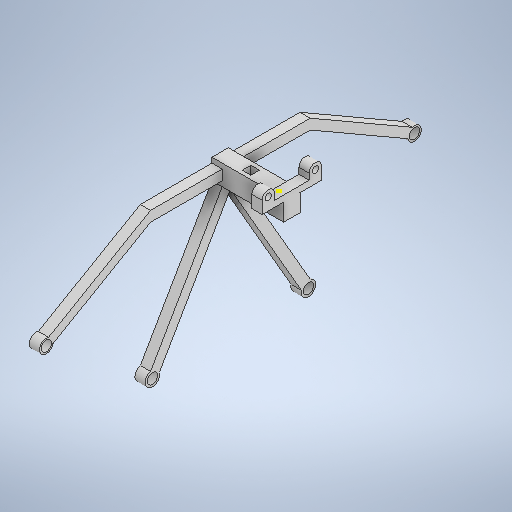
# Autodesk Inventor part: Pelvis proto1
Saved by Autodesk Inventor 2025.1 (Build 291241020, 241B)
## iProperties
Created: 2024-10-22
Part Number: Pelvis proto1
Material: Generic
Document SubType Name: Modeling
Designer: morte
Density: 1 g/cm^3
Appearance: Default
Author: morte
Autodesk Inventor part; units mm, degrees
ref_plane "YZ Plane" through (0, 0, 0) normal (1, 0, 0) x (0, 1, 0)
sketch "Sketch1" plane through (0, 0, 0) normal (1, 0, 0) x (0, 1, 0)
  line L0 (0, 0) -> (0, 8.5)
  line L1 (0, 14.5) -> (6, 14.5)
  line L2 (0, 0) -> (0, -8.5)
  line L3 (0, -14.5) -> (6, -14.5)
  line L4 (6, -14.5) -> (6, -8.5)
  line L5 (6, -8.5) -> (0, -8.5)
  line L6 (6, 14.5) -> (6, 8.5)
  line L7 (6, 8.5) -> (0, 8.5)
  line L8 (0, 14.5) -> (-3, 14.5)
  line L9 (-3, 14.5) -> (-3, -14.5)
  line L10 (-3, -14.5) -> (0, -14.5)
  line L11 (0, -8.5) -> (-3, -8.5)
  line L12 (0, 8.5) -> (-3, 8.5)
  line L13 (-3, 0) -> (-3, -5)
  dimension "d0" = 14.5
  dimension "d1" = 6
  dimension "d2" = 14.5
  dimension "d3" = 6
  dimension "d4" = 90
  dimension "d5" = 29
  dimension "d6" = 6
  dimension "d7" = 6
  dimension "d8" = 3
  dimension "d9" = 5
  constraints: 28 end point, 7 perpendicular, 4 point on line, 3 vertical, 1 collinear, 1 horizontal, 1 midpoint
  measures "d0" distance of L0.start L1.start
  measures "d1" distance of L1.start L1.end
  measures "d2" distance of L0.start L3.start
  measures "d3" distance of L3.start L3.end
  measures "d4" angle of L3 L2
  measures "d5" distance of L3.start L1.start
  measures "d6" distance of L3.end L4.end
  measures "d7" distance of L1.end L6.end
  measures "d8" distance of L1.start L8.end
  measures "d9" distance of L13.start L13.end
extrude "Extrusion1" add sketch "Sketch1" along normal mid plane 5
sketch "Sketch2" plane through (2.5, 0, 0) normal (1, 0, 0) x (0, 0, -1)
  line L0 (8.5, 0) -> (-8.5, 0) projected
  line L1 (0, 0) -> (-8.5, 0)
  line L2 (-8.5, 0) -> (-11.5, 0)
  line L3 (-14.5, 6) -> (-14.5, -3) projected
  line L4 (-11.5, 0) -> (-11.5, 3)
  line L5 (8.5, 0) -> (11.5, 0)
  line L6 (11.5, 0) -> (11.5, 3)
  circle A0 centre (-11.5, 3) radius 1.5
  circle A1 centre (11.5, 3) radius 1.5
  dimension "d14" = 3
  dimension "d15" = 3
  dimension "d16" = 3
  dimension "d17" = 3
  dimension "d18" = 3
  dimension "d19" = 3
  constraints: 10 end point, 3 perpendicular, 2 centre point, 2 coincident, 1 collinear, 1 horizontal
  measures "d14" distance of L0.end L2.end
  measures "d15" distance of L2.end L4.end
  measures "d16" distance of L0.start L5.end
  measures "d17" distance of L5.end L6.end
  measures "d18" diameter of A0
  measures "d19" diameter of A1
extrude "Extrusion2" cut sketch "Sketch2" against normal blind 10
sketch "Sketch3" plane through (-2.5, 0, 0) normal (-1, 0, 0) x (0, 0, 1)
  circle A0 centre (-11.5, 3) radius 1.5 projected
  circle A1 centre (-11.5, 3) radius 3
  line L0 (-14.5, 3) -> (-14.5, 7.7039)
  line L1 (-14.5, -3) -> (-14.5, 6) projected
  line L2 (-14.5, 7.7039) -> (-8.5, 7.7039)
  line L3 (-8.5, 7.7039) -> (-8.5, 3)
  circle A2 centre (11.5, 3) radius 1.5 projected
  circle A3 centre (11.5, 3) radius 3
  line L4 (8.5, 3) -> (8.5, 6.9796)
  line L5 (8.5, 6.9796) -> (14.5, 6.9796)
  line L6 (14.5, 6.9796) -> (14.5, 3)
  line L7 (14.5, 6) -> (14.5, -3) projected
  point P0 (0, 0)
  constraints: 12 end point, 4 point on circle, 2 centre point, 2 coincident, 2 perpendicular, 2 tangent, 1 collinear, 1 point on line, 1 vertical
extrude "Extrusion3" cut sketch "Sketch3" against normal through all contours A1 L0 L2 L3 | A3 L4 L5 L6
sketch "Sketch4" plane through (2.5, 0, 0) normal (1, 0, 0) x (0, 0, -1)
  line L0 (14.5, -3) -> (-14.5, -3) projected
  line L1 (0, -3) -> (4, -3)
  line L2 (0, -3) -> (-4, -3)
  line L3 (-4, -3) -> (-4, -1.5)
  line L4 (-4, -1.5) -> (4, -1.5)
  line L5 (4, -1.5) -> (4, -11.5)
  line L6 (4, -11.5) -> (-4, -11.5)
  line L7 (-4, -11.5) -> (-4, -1.5)
  point P0 (0, 0)
  dimension "d24" = 4
  dimension "d25" = 4
  dimension "d26" = 1.5
  dimension "d27" = 10
  dimension "d28" = 8
  constraints: 14 end point, 3 perpendicular, 3 point on line, 1 collinear, 1 midpoint
  measures "d24" distance of L1.start L1.end
  measures "d25" distance of L1.start L2.end
  measures "d26" distance of L2.end L3.end
  measures "d27" distance of L4.end L5.end
  measures "d28" distance of L5.end L6.end
extrude "Extrusion4" add sketch "Sketch4" against normal blind 35
sketch "Sketch5" plane through (2.5, -11.5, -4) normal (0, -1, 0) x (1, 0, 0)
  line L0 (0, -4.5) -> (0, 12.5) projected
  line L1 (0, 0) -> (-20, 0)
  line L2 (0, 0) -> (-35, 0) projected
  line L3 (-20, 0) -> (-20, 4)
  line L4 (0, 8) -> (-35, 8) projected
  line L5 (-22.1, 1.9) -> (-17.9, 1.9)
  line L6 (-17.9, 1.9) -> (-17.9, 6.1)
  line L7 (-17.9, 6.1) -> (-22.1, 6.1)
  line L8 (-22.1, 6.1) -> (-22.1, 1.9)
  line L9 (-22.1, 1.9) -> (-17.9, 6.1) construction
  line L10 (-17.9, 1.9) -> (-22.1, 6.1) construction
  point P0 (-2.5, 4)
  dimension "d31" = 20
  dimension "d32" = 4
  dimension "d132" = 4.2
  dimension "d133" = 4.2
  constraints: 16 end point, 2 midpoint, 2 parallel, 2 perpendicular, 2 point on line, 1 horizontal
  measures "d31" distance of L1.start L1.end
  measures "d32" distance of L1.end L3.end
  measures "d132" distance of L7.end L6.end
  measures "d133" distance of L5.end L6.end
extrude "Extrusion5" cut sketch "Sketch5" against normal through all
sketch "Sketch8" plane through (2.5, -11.5, 4) normal (0, 0, 1) x (1, 0, 0)
  point P0 (-2.5, 11.5)
sketch "Sketch12" plane through (-32.5, 0, 0) normal (-1, 0, 0) x (0, 0, 1)
  line L0 (4, -11.5) -> (4, -1.5) projected
  line L1 (4, -1.5) -> (-4, -1.5) projected
  line L2 (4, -1.5) -> (4, -4)
  line L3 (4, -3) -> (4, -11.5) projected
  line L4 (4, -4) -> (4, -9)
  line L5 (4, -9) -> (39, -9)
  line L6 (39, -9) -> (39, -4)
  line L7 (39, -4) -> (4, -4)
  point P0 (0, 0)
  dimension "d63" = 2.5
  dimension "d64" = 5
  dimension "d65" = 35
  dimension "d66" = 5
  constraints: 10 end point, 2 perpendicular, 2 point on line
  measures "d63" distance of L0.end L2.end
  measures "d64" distance of L2.end L4.end
  measures "d65" distance of L4.end L5.end
  measures "d66" distance of L5.end L6.end
extrude "Extrusion10" add sketch "Sketch12" against normal blind 5
sketch "Sketch13" plane through (-32.5, 0, 0) normal (-1, 0, 0) x (0, 0, 1)
  line L0 (4, -4) -> (39, -4) projected
  line L1 (39, -4) -> (94, -4) construction
  line L2 (39, -4) -> (39, -9) projected
  line L3 (39, -4) -> (4, -4) projected
  line L4 (39, -4) -> (88.7965, -32.75)
  line L5 (39, -4) -> (96.5, -4) construction
  line L6 (39, -9) -> (86.6314, -36.5)
  line L7 (39, -9) -> (94, -9) construction
  line L8 (86.6314, -36.5) -> (88.7965, -32.75)
  point P0 (0, 0)
  dimension "d95" = 30
  dimension "d96" = 30
  dimension "d108" = 55
  constraints: 12 end point, 3 horizontal, 2 equal length, 1 perpendicular
  measures "d95" angle of L4 L5
  measures "d96" angle of L6 L7
  measures "d108" distance of L2.end L6.end
extrude "Extrusion11" add sketch "Sketch13" against normal blind 5
sketch "Sketch14" plane through (-32.5, 0, 0) normal (-1, 0, 0) x (0, 0, 1)
  line L0 (-4, -1.5) -> (4, -1.5) projected
  line L1 (-4, -1.5) -> (-4, -4)
  line L2 (-4, -3) -> (-4, -1.5) projected
  line L3 (-4, -4) -> (-4, -9)
  line L4 (-4, -9) -> (-39, -9)
  line L5 (-39, -9) -> (-39, -4)
  line L6 (-39, -4) -> (-4, -4)
  point P0 (0, 0)
  dimension "d74" = 2.5
  dimension "d75" = 5
  dimension "d76" = 35
  constraints: 10 end point, 3 perpendicular, 1 collinear, 1 point on line
  measures "d74" distance of L0.start L1.end
  measures "d75" distance of L1.end L3.end
  measures "d76" distance of L3.end L4.end
extrude "Extrusion12" add sketch "Sketch14" against normal blind 5
sketch "Sketch15" plane through (-32.5, 0, 0) normal (-1, 0, 0) x (0, 0, 1)
  line L0 (-39, -4) -> (-4, -4) projected
  line L1 (-39, -4) -> (16, -4) construction
  line L2 (-39, -9) -> (-39, -4) projected
  line L3 (-39, -9) -> (-23.5212, -9) construction
  line L4 (-39, -9) -> (13.5, -9) construction
  line L5 (-39, -9) -> (-86.6314, -36.5)
  line L6 (-39, -9) -> (16, -9) construction
  line L7 (-39, -4) -> (-88.7965, -32.75)
  line L8 (-39, -4) -> (18.5, -4) construction
  line L9 (-86.6314, -36.5) -> (-88.7965, -32.75)
  point P0 (0, 0)
  dimension "d90" = 55
  dimension "d91" = 150
  dimension "d93" = 150
  constraints: 16 end point, 5 horizontal, 2 equal length, 1 point on line
  measures "d90" distance of L2.start L5.end
  measures "d91" angle of L5 L6
  measures "d93" angle of L7 L8
extrude "Extrusion13" add sketch "Sketch15" against normal blind 5
sketch "Sketch17" plane through (-32.5, 0, 0) normal (-1, 0, 0) x (0, 0, 1)
  line L0 (-86.6314, -36.5) -> (-39, -9) projected
  line L1 (-39, -4) -> (-88.7965, -32.75) projected
  line L2 (-86.6314, -36.5) -> (-88.7965, -32.75) projected
  line L3 (-86.6314, -36.5) -> (-87.7139, -34.6251)
  line L4 (-87.7139, -34.6251) -> (-89.879, -35.8751)
  circle A0 centre (-89.879, -35.8751) radius 2.5
  circle A1 centre (-89.879, -35.8751) radius 3.3071
  line L5 (88.7965, -32.75) -> (87.714, -34.6249)
  line L6 (86.6314, -36.5) -> (88.7965, -32.75) projected
  line L7 (87.714, -34.6249) -> (89.879, -35.8749)
  circle A2 centre (89.879, -35.8749) radius 2.5
  line L8 (39, -9) -> (86.6314, -36.5) projected
  circle A3 centre (89.879, -35.8749) radius 3.3072
  point P0 (0, 0)
  point P1 (-88.7964, -32.7501)
  dimension "d124" = 6.6145
  dimension "d101" = 2.165
  dimension "d102" = 2.5
  dimension "d106" = 2.165
  dimension "d107" = 2.5
  constraints: 8 end point, 4 coincident, 2 perpendicular, 2 point on line, 12 other
  measures "d101" distance of L0.start L3.end
  measures "d102" distance of L3.end L4.end
  measures "d106" distance of L5.start L5.end
  measures "d107" distance of L5.end L7.end
extrude "Extrusion14" add sketch "Sketch17" against normal blind 5
ref_plane "Work Plane3" through (2.5, -11.5, 4) normal (0, -0.8660254, 0.5) x (-1, 0, 0)
sketch "Sketch18" plane through (2.5, -11.5, 4) normal (0, -0.8660254, 0.5) x (-1, 0, 0)
  line L0 (0, 0) -> (35, 0) projected
  line L1 (35, 0) -> (30, 0)
  line L2 (30, 0) -> (30, 5)
  line L3 (30, 5) -> (35, 5)
  line L4 (30, 5) -> (35, 5) construction
  line L5 (35, 5) -> (35, 0)
  point P0 (2.5, -2.2859)
  dimension "d110" = 5
  dimension "d111" = 5
  dimension "d112" = 5
  dimension "d113" = 0
  constraints: 10 end point, 2 horizontal, 1 collinear, 1 perpendicular, 1 point on line
  measures "d110" distance of L0.end L1.end
  measures "d111" distance of L1.end L2.end
  measures "d112" distance of L2.end L3.end
  measures "d113" distance between parallel lines of L3 L4
extrude "Extrusion15" add sketch "Sketch18" along normal blind 70
ref_plane "Work Plane4" through (2.5, -11.5, -4) normal (0, -0.8660254, -0.5) x (-1, 0, 0)
sketch "Sketch19" plane through (2.5, -11.5, -4) normal (0, -0.8660254, -0.5) x (-1, 0, 0)
  line L0 (35, 0) -> (35, -6.9282) projected
  line L1 (35, 0) -> (30, 0)
  line L2 (0, 0) -> (35, 0) projected
  line L3 (30, 0) -> (30, -5)
  line L4 (30, -5) -> (35, -5)
  line L5 (35, -5) -> (35, 0)
  point P0 (2.5, 2.2859)
  dimension "d117" = 5
  dimension "d118" = 5
  dimension "d119" = 90
  constraints: 8 end point, 3 perpendicular, 1 point on line
  measures "d117" distance of L0.start L1.end
  measures "d118" distance of L1.end L3.end
  measures "d119" angle of L3 L1
extrude "Extrusion16" add sketch "Sketch19" along normal blind 70
sketch "Sketch20" plane through (-27.5, -72.1218, 39) normal (1, 0, 0) x (0, -0.5, -0.8660254)
  line L0 (0, 70) -> (0, 0) projected
  line L1 (6.9282, 74) -> (0, 70)
  line L2 (6.9282, 74) -> (2.6782, 81.3612) projected
  line L3 (0, 70) -> (4.6188, 70) projected
  line L4 (6.9282, 74) -> (67.55, 39) projected
  line L5 (4.6188, 70) -> (6.9282, 74)
  point P0 (-2.2859, 81.9593)
  constraints: 4 end point, 2 perpendicular
extrude "Extrusion17" add sketch "Sketch20" against normal blind 5
sketch "Sketch21" plane through (-27.5, -11.5, 4) normal (1, 0, 0) x (0, 0, -1)
  line L0 (-35, -60.6218) -> (-30.6699, -63.1218) projected
  line L1 (-30.6699, -63.1218) -> (-32.8349, -61.8718)
  line L2 (-32.8349, -61.8718) -> (-34.0849, -64.0368)
  line L3 (-32.8349, -61.8718) -> (-30.3349, -61.8718) construction
  circle A0 centre (-34.0849, -64.0368) radius 2.5
  arc A1 (-35, -60.6218) -> (-30.6699, -63.1218) centre (-34.0849, -64.0368) ccw
  line L4 (43, -60.6218) -> (38.6699, -63.1218) projected
  line L5 (43, -60.6218) -> (40.8349, -61.8718)
  line L6 (40.8349, -61.8718) -> (42.0849, -64.0368)
  circle A2 centre (42.0849, -64.0368) radius 2.5
  line L7 (4, -3.0718) -> (38.6699, -63.1218) projected
  arc A3 (38.6699, -63.1218) -> (43, -60.6218) centre (42.0849, -64.0368) ccw
  point P0 (4, 11.5)
  dimension "d125" = 2.5
  dimension "d126" = 2.5
  dimension "d127" = 120
  dimension "d129" = 2.5
  constraints: 12 end point, 4 coincident, 4 point on circle, 2 centre point, 2 midpoint, 1 equal length, 1 horizontal, 1 perpendicular, 1 point on line, 6 other
  measures "d125" distance of L0.end L1.end
  measures "d126" distance of L1.end L2.end
  measures "d127" angle of L2 L3
  measures "d129" distance of L4.start L5.end
extrude "Extrusion18" add sketch "Sketch21" against normal blind 5
body "Solid1"
